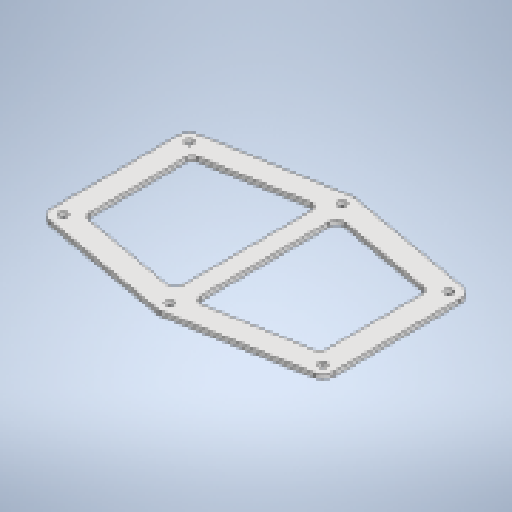
# Autodesk Inventor part: podstawa
Saved by Autodesk Inventor 2023 (Build 270158000, 158)
## iProperties
Created: 2024-10-16
Part Number: podstawa
Material: Ogólny
Document SubType Name: Modeling
Designer: kamil
Density: 1 g/cm^3
Appearance: Domyślna
Author: kamil
Autodesk Inventor part; units mm, degrees
ref_plane "YZ Plane" through (0, 0, 0) normal (1, 0, 0) x (0, 1, 0)
ref_plane "XZ Plane" through (0, 0, 0) normal (0, 1, 0) x (-1, 0, 0)
ref_plane "XY Plane" through (0, 0, 0) normal (0, 0, 1) x (1, 0, 0)
sketch "Szkic1" plane through (0, 0, 0) normal (0, 1, 0) x (-1, 0, 0)
  line L0 (0, 0) -> (0, -75) construction
  line L1 (-56.5, -37.5) -> (56.5, -37.5) construction
  line L2 (56.5, -10) -> (56.5, -65) construction
  line L3 (-56.5, -10) -> (-56.5, -65) construction
  circle A0 centre (56.5, -10) radius 5
  circle A1 centre (56.5, -65) radius 5
  circle A2 centre (0, 0) radius 5
  circle A3 centre (0, -75) radius 5
  circle A4 centre (-56.5, -10) radius 5
  circle A5 centre (-56.5, -65) radius 5
  line L4 (0.8714, 4.9235) -> (57.3714, -5.0765)
  line L5 (57.3714, -69.9235) -> (0.8714, -79.9235)
  line L6 (-0.8714, -79.9235) -> (-57.3714, -69.9235)
  line L7 (-57.3714, -5.0765) -> (-0.8714, 4.9235)
  line L8 (-61.5, -10) -> (-61.5, -65)
  line L9 (61.5, -10) -> (61.5, -65)
  point P0 (0, -37.5)
  point P1 (0, -37.5)
  dimension "d0" = 75
  dimension "d1" = 113
  dimension "d2" = 55
  dimension "d3" = 55
  dimension "d4" = 10
  dimension "d5" = 10
  dimension "d6" = 10
  dimension "d7" = 10
  dimension "d8" = 10
  dimension "d9" = 10
  constraints: 20 end point, 16 coincident, 12 point on circle, 12 tangent, 6 centre point, 4 midpoint, 3 vertical, 2 vertical alignment, 1 horizontal
  measures "d0" distance of L0.start L0.end
  measures "d1" distance of L1.start L1.end
  measures "d2" distance of L2.start L2.end
  measures "d3" distance of L3.start L3.end
  measures "d4" diameter of A0
  measures "d5" diameter of A1
  measures "d6" diameter of A2
  measures "d7" diameter of A3
  measures "d8" diameter of A4
  measures "d9" diameter of A5
extrude "Wyciągnięcie proste1" add sketch "Szkic1" along normal blind 2
sketch "Szkic2" plane through (0, 2, 0) normal (0, 1, 0) x (1, 0, 0)
  arc A0 (-0.8714, -4.9235) -> (0.8714, -4.9235) centre (0, 0) ccw projected
  arc A1 (0.8714, 79.9235) -> (-0.8714, 79.9235) centre (0, 75) ccw projected
  arc A2 (61.5, 65) -> (57.3714, 69.9235) centre (56.5, 65) ccw projected
  arc A3 (57.3714, 5.0765) -> (61.5, 10) centre (56.5, 10) ccw projected
  arc A4 (-61.5, 10) -> (-57.3714, 5.0765) centre (-56.5, 10) ccw projected
  arc A5 (-57.3714, 69.9235) -> (-61.5, 65) centre (-56.5, 65) ccw projected
hole "Otwór1" at (-56.5, 2, -65) at (-56.5, 2, -10) at (0, 2, 0) at (56.5, 2, -10) at (0, 2, -75) at (56.5, 2, -65) direction (0, -1, 0) diameter 3.5 depth 8
sketch "Szkic3" plane through (0, 2, 0) normal (0, 1, 0) x (1, 0, 0)
  circle A0 centre (0, 75) radius 1.75 projected
  circle A1 centre (0, 0) radius 1.75 projected
  circle A2 centre (-56.5, 65) radius 1.75 projected
  circle A3 centre (-56.5, 10) radius 1.75 projected
  circle A4 centre (56.5, 10) radius 1.75 projected
  circle A5 centre (56.5, 65) radius 1.75 projected
  arc A6 (-61.5, 10) -> (-57.3714, 5.0765) centre (-56.5, 10) ccw projected
  line L0 (-57.3714, 5.0765) -> (-0.8714, -4.9235) projected
  arc A7 (-0.8714, -4.9235) -> (0.8714, -4.9235) centre (0, 0) ccw projected
  line L1 (0.8714, -4.9235) -> (57.3714, 5.0765) projected
  arc A8 (57.3714, 5.0765) -> (61.5, 10) centre (56.5, 10) ccw projected
  line L2 (61.5, 10) -> (61.5, 65) projected
  arc A9 (61.5, 65) -> (57.3714, 69.9235) centre (56.5, 65) ccw projected
  line L3 (57.3714, 69.9235) -> (0.8714, 79.9235) projected
  arc A10 (0.8714, 79.9235) -> (-0.8714, 79.9235) centre (0, 75) ccw projected
  line L4 (-0.8714, 79.9235) -> (-57.3714, 69.9235) projected
  arc A11 (-57.3714, 69.9235) -> (-61.5, 65) centre (-56.5, 65) ccw projected
  line L5 (-61.5, 65) -> (-61.5, 10) projected
  line L6 (0, 5.0777) -> (-51.5, 14.1928)
  line L7 (-51.5, 14.1928) -> (-51.5, 60.8072)
  line L8 (-51.5, 60.8072) -> (0, 69.9223)
  line L9 (0, 69.9223) -> (51.5, 60.8072)
  line L10 (51.5, 60.8072) -> (51.5, 14.1928)
  line L11 (51.5, 14.1928) -> (0, 5.0777)
  circle A12 centre (0, 0) radius 1.75 projected
  circle A13 centre (0, 75) radius 1.75 projected
  line L12 (0, 0) -> (0, 75) construction
  line L13 (4.0221, 0) -> (4.0221, 75)
  line L14 (-4.0221, 75) -> (-4.0221, 0)
  arc A14 (-4.0221, 0) -> (4.0221, 0) centre (0, 0) ccw
  arc A15 (4.0221, 75) -> (-4.0221, 75) centre (0, 75) ccw
  point P0 (0, 37.5)
  point P1 (4.0221, 69.2104)
  point P2 (4.0221, 5.7896)
  point P3 (-4.0221, 5.7896)
  point P4 (-4.0221, 69.2104)
  dimension "d19" = 10
  constraints: 20 end point, 4 point on circle, 4 tangent, 2 centre point, 1 midpoint, 1 parallel, 5 other
  measures "d19" distance between parallel lines of L0 L6
extrude "Wyciągnięcie proste2" cut sketch "Szkic3" against normal through all contours L6 L7 L8 L14 | L13 L9 L10 L11
fillet "Zaokrąglenie1" radius 3 8 edges at (-51.5, 1, -60.8072) (-51.5, 1, -14.1928) (-4.0221, 1, -5.7896) (4.0221, 1, -5.7896) (-4.0221, 1, -69.2104) (4.0221, 1, -69.2104) (51.5, 1, -60.8072) (51.5, 1, -14.1928)
